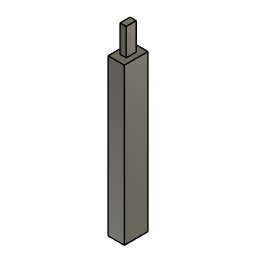
hobby-motor-with-encoder-v1 (Autodesk Fusion 360 design; units mm, degrees)
Autodesk Fusion 360 part; units mm, degrees
sketch "Sketch1" plane through (0, 0, 0) normal (0, 0, 1) x (1, 0, 0)
  line L0 (21, 6) -> (30, 6)
  line L1 (30, 6) -> (30, -7)
  line L2 (30, -7) -> (21, -7)
  line L3 (21, -7) -> (21, 6)
  constraint horizontal L0
  constraint vertical L1
  constraint horizontal L2
  constraint vertical L3
extrude "Extrude1" add sketch "Sketch1" along normal blind 86
hole "Hole1" at (25.6586, -0.5801, 0) direction (0, 0, 1) diameter 5.5 depth 15 tip angle 118
sketch "Sketch2" plane through (0, 0, 86) normal (0, 0, 1) x (-1, 0, 0)
  line L0 (-21, 7) -> (-30, 7)
  line L1 (-30, 7) -> (-30, -6)
  line L2 (-30, -6) -> (-21, -6)
  line L3 (-21, -6) -> (-21, 7)
  line L4 (-27, 3) -> (-23.6227, 3)
  line L5 (-23.6227, 3) -> (-23.6227, -2.5485)
  line L6 (-23.6227, -2.5485) -> (-27, -2.5485)
  line L7 (-27, -2.5485) -> (-27, 3)
  constraint horizontal L4
  constraint vertical L5
  constraint horizontal L6
  constraint vertical L7
extrude "Extrude2" add sketch "Sketch2" along normal blind 15 contours L4 L5 L6 L7
component "part_object_id_2" placed x (1, 0, 0) y (0, 1, 0) z (0, 0, 1) at (0, 0, 0)
